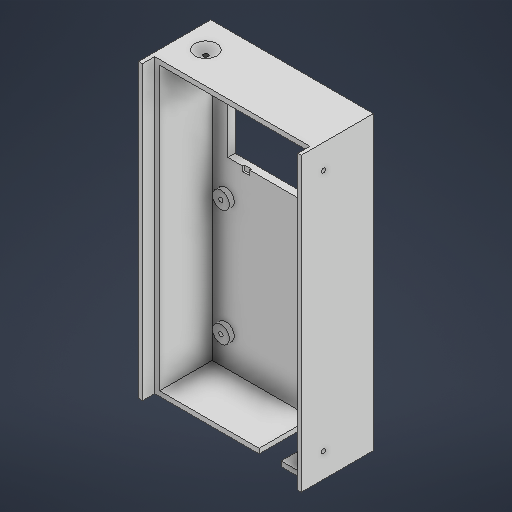
# Autodesk Inventor part: Bottom_Shell
Saved by Autodesk Inventor 2027 (Build 310192000, 192)
## iProperties
Created: 2026-03-03
Part Number: Bottom_Shell
Material: Generic
Document SubType Name: Modeling
Designer: kjedr
Density: 1 g/cm^3
Appearance: Default
Author: kjedr
Autodesk Inventor part; units mm, degrees
ref_plane "YZ Plane" through (0, 0, 0) normal (1, 0, 0) x (0, 1, 0)
ref_plane "XZ Plane" through (0, 0, 0) normal (0, 1, 0) x (-1, 0, 0)
ref_plane "XY Plane" through (0, 0, 0) normal (0, 0, 1) x (1, 0, 0)
sketch "Sketch1" plane through (0, 0, 0) normal (0, 0, 1) x (1, 0, 0)
  line L0 (0, 0) -> (80.8355, 0)
  line L1 (80.8355, 0) -> (80.8355, 152.4)
  line L2 (80.8355, 152.4) -> (0, 152.4)
  line L3 (0, 152.4) -> (0, 0)
  dimension "d82" = 80.8355
  dimension "d90" = 152.4
  constraints: 8 end point, 3 perpendicular
  measures "d82" distance of L1.end L2.end
  measures "d90" distance of L2.end L0.start
extrude "Extrusion1" add sketch "Sketch1" along normal blind 22.86
sketch "Sketch2" plane through (0, 0, 22.86) normal (0, 0, 1) x (1, 0, 0)
  line L0 (2.54, 2.54) -> (78.2955, 2.54)
  line L1 (78.2955, 2.54) -> (78.2955, 149.86)
  line L2 (78.2955, 149.86) -> (2.54, 149.86)
  line L3 (2.54, 149.86) -> (2.54, 2.54)
  line L4 (0, 152.4) -> (0, 0)
  line L5 (0, 0) -> (80.8355, 0)
  line L6 (80.8355, 0) -> (80.8355, 152.4)
  line L7 (80.8355, 152.4) -> (0, 152.4)
  line L8 (0, 152.4) -> (0, 0) projected
  line L9 (0, 0) -> (80.8355, 0) projected
  point P0 (80.8355, 76.2)
  point P1 (0, 76.2)
  point P2 (40.4177, 0)
  dimension "d83" = 152.4
  dimension "d85" = 80.8355
  dimension "d86" = 2.54
  dimension "d87" = 2.54
  dimension "d88" = 2.54
  dimension "d89" = 2.54
  constraints: 16 end point, 5 midpoint, 5 perpendicular
  measures "d83" distance of L4.start L4.end
  measures "d85" distance of L6.end L4.start
  measures "d86" horizontal distance of L2.end L4.start
  measures "d87" horizontal distance of L2.end L4.start
  measures "d88" horizontal distance of L4.end L0.start
  measures "d89" horizontal distance of L5.end L0.end
extrude "Extrusion2" cut sketch "Sketch2" against normal blind 19.05 contours L3 L2 L1 L0
sketch "Sketch6" plane through (0, 0, 3.81) normal (0, 0, 1) x (1, 0, 0)
  line L0 (5.1487, 87.2258) -> (75.6867, 87.2258) construction
  line L1 (75.6867, 87.2258) -> (75.6867, 3.2258) construction
  line L2 (75.6867, 3.2258) -> (5.1487, 3.2258) construction
  line L3 (5.1487, 3.2258) -> (5.1487, 87.2258) construction
  circle A0 centre (9.6205, 79.9318) radius 1.6 construction
  circle A1 centre (71.2409, 79.9318) radius 1.6 construction
  circle A2 centre (9.6205, 19.2258) radius 1.6 construction
  circle A3 centre (71.2409, 19.2258) radius 1.6 construction
  line L4 (2.54, 149.86) -> (78.2955, 149.86) projected
  line L5 (0, 0) -> (80.8355, 0) projected
  line L6 (78.2955, 2.54) -> (2.54, 2.54) projected
  circle A4 centre (9.6205, 79.9318) radius 4.445
  circle A5 centre (71.2409, 79.9318) radius 4.445
  circle A6 centre (9.6205, 19.2258) radius 4.445
  circle A7 centre (71.2409, 19.2258) radius 4.445
  point P0 (40.4177, 87.2258)
  point P1 (40.4177, 149.86)
  point P2 (3.175, 0)
  point P3 (77.6605, 0)
  point P4 (2.54, 2.54)
  point P5 (14.1287, 30.2258)
  point P6 (46.6867, 15.7258)
  point P7 (60.2637, 3.2258)
  point P8 (80.8355, 12.6941)
  dimension "d18" = 70.538
  dimension "d19" = 84
  dimension "d30" = 3.2
  dimension "d31" = 60.706
  dimension "d32" = 61.6204
  dimension "d33" = 16
  dimension "d34" = 4.4458
  dimension "d36" = 0.6858
  dimension "d37" = 27
  dimension "d38" = 8.98
  dimension "d39" = 12.5
  dimension "d40" = 29
  dimension "d41" = 15.423
  dimension "d69" = 8.89
  dimension "d70" = 8.89
  dimension "d71" = 8.89
  dimension "d72" = 8.89
  constraints: 8 centre point, 8 end point, 4 coincident, 3 equal radius, 3 vertical alignment, 2 horizontal alignment, 2 midpoint, 2 parallel, 1 horizontal, 1 perpendicular, 1 point on line, 1 other
  measures "d18" distance of L1.end L2.end
  measures "d19" distance of L0.end L1.end
  measures "d30" diameter of A0
  measures "d31" distance of A2.centre A0.centre
  measures "d32" distance of A3.centre A2.centre
  measures "d33" distance from line of L2 A3.centre
  measures "d34" distance from line of L1 A3.centre
  measures "d37" distance from line of L2 point (14.129, 30.226)
  measures "d38" distance from line of L3 point (14.129, 30.226)
  measures "d39" distance from line of L2 point (46.687, 15.726)
  measures "d40" distance from line of L1 point (46.687, 15.726)
  measures "d41" distance from line of L1 point (60.264, 3.226)
  measures "d69" diameter of A4
  measures "d70" diameter of A5
  measures "d71" diameter of A6
  measures "d72" diameter of A7
extrude "Extrusion7" add sketch "Sketch6" along normal blind 2.54
sketch "Sketch15" plane through (9.6205, 79.9318, 6.35) normal (0, 0, 1) x (1, 0, 0)
  circle A0 centre (0, 0) radius 4.445 projected
  circle A1 centre (61.6204, 0) radius 4.445 projected
  circle A2 centre (61.6204, -60.706) radius 4.445 projected
  circle A3 centre (0, -60.706) radius 4.445 projected
  point P0 (-9.6205, -79.9318)
  point P1 (61.6204, -60.706)
  point P2 (0, -60.706)
  constraints: 4 coincident
hole "Hole3" at (9.6205, 79.9318, 6.35) at (71.2409, 79.9318, 6.35) at (71.2409, 19.2258, 6.35) at (9.6205, 19.2258, 6.35) direction (0, 0, -1) diameter 2.286 depth 6.35
sketch "Sketch16" plane through (0, 0, 3.81) normal (0, 0, 1) x (1, 0, 0)
  line L0 (10.6608, 147.32) -> (70.5655, 147.32)
  line L1 (70.5655, 147.32) -> (70.5655, 98.3851)
  line L2 (70.5655, 98.3851) -> (10.6608, 98.3851)
  line L3 (10.6608, 98.3851) -> (10.6608, 147.32)
  line L4 (2.54, 149.86) -> (78.2955, 149.86) projected
  point P0 (0, 0)
  dimension "d150" = 48.9349
  dimension "d151" = 59.9047
  dimension "d152" = 2.54
  constraints: 8 end point, 2 parallel, 1 horizontal, 1 perpendicular
  measures "d150" distance of L0.end L1.end
  measures "d151" distance of L0.start L0.end
  measures "d152" distance between parallel lines of L4 L0
extrude "Extrusion8" cut sketch "Sketch16" against normal blind 25.4
sketch "Sketch17" plane through (2.54, 149.86, 22.86) normal (0, -1, 0) x (1, 0, 0)
  circle A0 centre (7.709, -8.0113) radius 1.27
  point P0 (-2.54, -22.86)
  dimension "d93" = 2.54
  constraints: 1 centre point
  measures "d93" diameter of A0
extrude "Extrusion9" cut sketch "Sketch17" along normal blind 25.4 and the other way blind 12.7 draft 60
sketch "Sketch18" plane through (10.6608, 98.3851, 3.81) normal (0, 1, 0) x (1, 0, 0)
  line L0 (59.9047, 0) -> (0, 0) projected
  line L1 (7.9345, 0) -> (11.287, 0)
  line L2 (11.287, 0) -> (11.287, 0.9229)
  line L3 (11.287, 0.9229) -> (7.9345, 0.9229)
  line L4 (7.9345, 0.9229) -> (7.9345, 0)
  line L5 (45.7582, 0) -> (49.8968, 0)
  line L6 (49.8968, 0) -> (49.8968, 0.9229)
  line L7 (49.8968, 0.9229) -> (45.7582, 0.9229)
  line L8 (45.7582, 0.9229) -> (45.7582, 0)
  point P0 (-10.6608, 3.81)
  point P1 (11.287, 0)
  constraints: 16 end point, 4 parallel, 3 point on line, 2 horizontal, 2 perpendicular
extrude "Extrusion10" cut sketch "Sketch18" against normal blind 2.54
sketch "Sketch19" plane through (0, 0, 3.81) normal (0, 0, 1) x (1, 0, 0)
  point P0 (0, 0)
sketch "Sketch23" plane through (0, 0, 0) normal (0, 0, -1) x (-1, 0, 0)
  line L0 (-84.6455, 152.4) -> (3.81, 152.4)
  line L1 (3.81, 152.4) -> (3.81, 0)
  line L2 (3.81, 0) -> (-84.6455, 0)
  line L3 (-84.6455, 0) -> (-84.6455, 152.4)
  line L4 (0, 0) -> (-80.8355, 0) projected
  line L5 (-80.8355, 152.4) -> (0, 152.4) projected
  line L6 (-80.8355, 0) -> (-80.8355, 152.4) projected
  line L7 (0, 152.4) -> (0, 0) projected
  point P0 (0, 152.4)
  dimension "d109" = 0
  dimension "d110" = 0
  dimension "d111" = 3.81
  dimension "d112" = 3.81
  constraints: 8 end point, 2 parallel, 1 horizontal, 1 perpendicular
  measures "d109" distance between parallel lines of L4 L2
  measures "d110" distance between parallel lines of L5 L0
  measures "d111" distance between parallel lines of L3 L6
  measures "d112" distance between parallel lines of L7 L1
extrude "Extrusion12" add sketch "Sketch23" against normal blind 29.21 contours L0 L6 L2 L3 | L0 L1 L2 L7
sketch "Sketch24" plane through (84.6455, 0, 0) normal (1, 0, 0) x (0, 0, -1)
  line L0 (-29.21, 0) -> (-29.21, 152.4) projected
  line L1 (0, 152.4) -> (-29.21, 152.4) projected
  line L2 (0, 0) -> (-29.21, 0) projected
  point P0 (-26.035, 12.7)
  point P1 (-26.035, 139.7)
  dimension "d115" = 3.175
  dimension "d116" = 12.7
  dimension "d117" = 12.7
  dimension "d118" = 3.175
  measures "d115" distance from line of L0 point (-26.035, 139.7)
  measures "d116" distance from line of L1 point (-26.035, 139.7)
  measures "d117" distance from line of L2 point (-26.035, 12.7)
  measures "d118" distance from line of L0 point (-26.035, 12.7)
hole "Hole5" at (84.6455, 139.7, 26.035) at (84.6455, 12.7, 26.035) direction (-1, 0, 0) diameter 2.286 end through all
sketch "Sketch25" plane through (-3.81, 0, 0) normal (0, -1, 0) x (1, 0, 0)
  line L0 (3.81, 22.86) -> (84.6455, 22.86) projected
  line L1 (58.3565, 22.86) -> (69.7865, 22.86)
  line L2 (69.7865, 22.86) -> (69.7865, 7.62)
  line L3 (69.7865, 7.62) -> (58.3565, 7.62)
  line L4 (58.3565, 7.62) -> (58.3565, 22.86)
  line L5 (88.4555, 0) -> (88.4555, 29.21) projected
  point P0 (3.81, 0)
  point P1 (69.7865, 15.24)
  point P2 (64.0715, 22.86)
  point P3 (64.0715, 7.62)
  point P4 (44.2278, 22.86)
  dimension "d126" = 11.43
  dimension "d127" = 15.24
  dimension "d129" = 19.8438
  constraints: 8 end point, 4 midpoint, 2 parallel, 1 horizontal, 1 perpendicular, 1 point on line
  measures "d126" distance from line of point (69.786, 15.24) L4
  measures "d127" distance from line of point (64.071, 22.86) L3
  measures "d129" horizontal distance of point (44.228, 22.86) point (64.071, 7.62)
extrude "Extrusion13" cut sketch "Sketch25" against normal up to surface (2.54 mm away)
sketch "Sketch26" plane through (-3.81, 0, 0) normal (0, -1, 0) x (1, 0, 0)
  line L0 (0, 29.21) -> (3.81, 29.21) projected
  line L1 (3.556, 29.21) -> (84.8995, 29.21)
  line L2 (84.8995, 29.21) -> (84.8995, 22.86)
  line L3 (84.8995, 22.86) -> (3.556, 22.86)
  line L4 (3.556, 22.86) -> (3.556, 29.21)
  line L5 (3.81, 22.86) -> (58.3565, 22.86) projected
  line L6 (3.81, 22.86) -> (3.81, 29.21) projected
  line L7 (84.6455, 22.86) -> (84.6455, 29.21) projected
  line L8 (3.81, 29.21) -> (84.6455, 29.21)
  line L9 (84.6455, 29.21) -> (84.6455, 22.86)
  line L10 (84.6455, 22.86) -> (3.81, 22.86)
  line L11 (3.81, 22.86) -> (3.81, 29.21)
  point P0 (3.81, 0)
  point P1 (84.8995, 26.035)
  dimension "d132" = 0
  dimension "d133" = 0.254
  dimension "d134" = 0.254
  constraints: 16 end point, 4 parallel, 2 horizontal, 2 perpendicular, 1 midpoint, 1 point on line
  measures "d132" distance between parallel lines of L5 L3
  measures "d133" distance between parallel lines of L6 L4
  measures "d134" distance from line of L7 point (84.899, 26.035)
extrude "Extrusion14" cut sketch "Sketch26" against normal through all contours L0 L6 L3 L4 | L1 L2 L3 L7
sketch "Sketch27" plane through (-3.81, 0, 0) normal (0, -1, 0) x (1, 0, 0)
  line L0 (0, 29.21) -> (1.778, 29.21)
  line L1 (1.778, 29.21) -> (1.778, 0)
  line L2 (1.778, 0) -> (0, 0)
  line L3 (0, 0) -> (0, 29.21)
  line L4 (3.556, 22.86) -> (3.556, 29.21) projected
  line L5 (88.4555, 0) -> (88.4555, 29.21) projected
  line L6 (88.4555, 0) -> (0, 0) projected
  line L7 (88.4555, 29.21) -> (86.6775, 29.21)
  line L8 (86.6775, 29.21) -> (86.6775, 0)
  line L9 (86.6775, 0) -> (88.4555, 0)
  line L10 (88.4555, 0) -> (88.4555, 29.21)
  point P0 (3.81, 0)
  point P1 (0.889, 0)
  dimension "d137" = 1.778
  dimension "d138" = 1.778
  dimension "d139" = 0
  constraints: 16 end point, 4 parallel, 2 horizontal, 2 perpendicular, 1 midpoint, 1 point on line
  measures "d137" distance between parallel lines of L4 L1
  measures "d138" distance of L9.end L8.end
  measures "d139" distance from line of L6 point (0.889, 0)
extrude "Extrusion15" cut sketch "Sketch27" against normal through all
sketch "Sketch28" plane through (0, 0, 22.86) normal (0, 0, 1) x (1, 0, 0)
  line L0 (-0.254, 152.4) -> (81.0895, 152.4) projected
  line L1 (82.8675, 0) -> (-2.032, 0) projected
  line L2 (-0.254, 152.4) -> (81.0895, 152.4)
  line L3 (81.0895, 152.4) -> (81.0895, 0)
  line L4 (81.0895, 0) -> (-0.254, 0)
  line L5 (-0.254, 0) -> (-0.254, 152.4)
  line L6 (81.0895, 152.4) -> (81.0895, 0) projected
  line L7 (2.54, 149.86) -> (78.2955, 149.86) projected
  line L8 (78.2955, 149.86) -> (78.2955, 2.54) projected
  line L9 (2.54, 149.86) -> (78.2955, 149.86)
  line L10 (78.2955, 149.86) -> (78.2955, 2.54)
  line L11 (78.2955, 2.54) -> (2.54, 2.54)
  line L12 (2.54, 2.54) -> (2.54, 149.86)
  line L13 (54.5465, 2.54) -> (2.54, 2.54) projected
  line L14 (54.5465, 0) -> (54.5465, 2.54) projected
  line L15 (54.5465, 2.54) -> (54.5465, 0)
  line L16 (65.9765, 0) -> (65.9765, 2.54) projected
  line L17 (65.9765, 0) -> (65.9765, 2.54)
  line L18 (78.2955, 2.54) -> (2.54, 2.54) projected
  point P0 (0, 0)
  point P1 (-0.254, 0)
  dimension "d142" = 0
  constraints: 20 end point, 5 equal length, 3 perpendicular, 2 horizontal, 2 point on line
  measures "d142" distance between parallel lines of L6 L3
extrude "Extrusion16" add sketch "Sketch28" along normal blind 8.4667 contours L0 L3 L1 L16 L11 L8 L7 L12 L14 L5
sketch "Sketch29" plane through (0, 0, 29.21) normal (0, 0, 1) x (1, 0, 0)
  line L0 (-2.032, 152.4) -> (82.8675, 152.4) projected
  line L1 (-2.032, 152.4) -> (0, 152.4)
  line L2 (0, 152.4) -> (0, 0)
  line L3 (0, 0) -> (-2.032, 0)
  line L4 (-2.032, 0) -> (-2.032, 152.4)
  line L5 (82.8675, 0) -> (82.8675, 152.4) projected
  line L6 (81.0895, 0) -> (81.0895, 152.4) projected
  line L7 (82.8675, 152.4) -> (81.0895, 152.4)
  line L8 (81.0895, 152.4) -> (81.0895, 0)
  line L9 (81.0895, 0) -> (82.8675, 0)
  line L10 (82.8675, 0) -> (82.8675, 152.4)
  constraints: 16 end point, 4 parallel, 2 horizontal, 2 perpendicular
extrude "Extrusion17" add sketch "Sketch29" along normal blind 8.4667
sketch "Sketch30" plane through (0, 0, 3.81) normal (0, 0, 1) x (1, 0, 0)
  line L0 (10.6608, 147.32) -> (70.5655, 147.32) projected
  line L1 (70.5655, 147.32) -> (70.5655, 98.3851) projected
  point P0 (0, 0)
  point P1 (53.6723, 150.7878)
  point P2 (57.4821, 140.1387)
  dimension "d154" = 3.4678
  dimension "d155" = 16.8932
  constraints: 1 other
  measures "d155" distance from line of L1 point (53.672, 150.788)
sketch "Sketch31" plane through (0, 0, 0) normal (0, 0, -1) x (-1, 0, 0)
  line L0 (-70.5655, 147.32) -> (-10.6608, 147.32) projected
  line L1 (-70.5655, 98.3851) -> (-70.5655, 147.32) projected
  point P0 (0, 0)
  point P1 (-53.6723, 150.7878)
  dimension "d156" = 3.4678
  dimension "d157" = 16.8932
  measures "d156" distance from line of L0 point (-53.672, 150.788)
  measures "d157" distance from line of L1 point (-53.672, 150.788)
hole "Hole6" at (53.6723, 150.7878, 0) direction (0, 0, 1) diameter 2.286 depth 12.7
body "Solid1"
